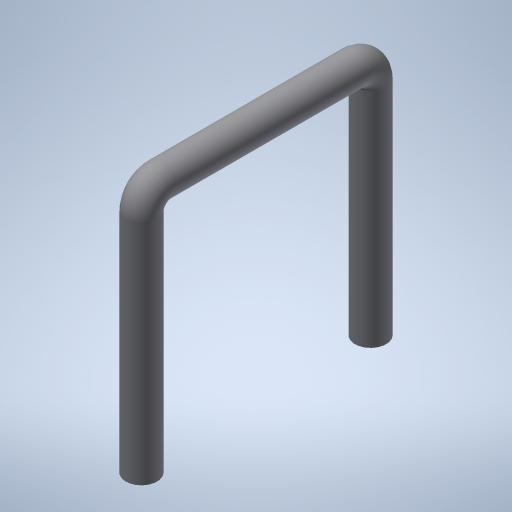
# Autodesk Inventor part: BRAZOS BAILARINA
Saved by Autodesk Inventor 2024 (Build 280153000, 153)
## iProperties
Created: 2025-03-28
Part Number: BRAZOS BAILARINA
Material: Generic
Document SubType Name: Modeling
Designer: usuario
Density: 1 g/cm^3
Appearance: Default
Author: usuario
Autodesk Inventor part; units mm, degrees
ref_plane "YZ Plane" through (0, 0, 0) normal (1, 0, 0) x (0, 1, 0)
ref_plane "XZ Plane" through (0, 0, 0) normal (0, 1, 0) x (-1, 0, 0)
ref_plane "XY Plane" through (0, 0, 0) normal (0, 0, 1) x (1, 0, 0)
sketch "Boceto1" plane through (0, 0, 0) normal (1, 0, 0) x (0, 1, 0)
  line L0 (0, 8.3393) -> (23, 8.3393)
  line L1 (25, 6.3393) -> (25, -13.2007)
  line L2 (23, -15.2007) -> (0.45, -15.2007)
  arc A0 (25, 6.3393) -> (23, 8.3393) centre (23, 6.3393) ccw
  arc A1 (23, -15.2007) -> (25, -13.2007) centre (23, -13.2007) ccw
  line L3 (0, 13.6272) -> (0, -20.4886) projected
  point P0 (0, 0)
  point P1 (25, 8.3393)
  point P2 (25, -15.2007)
  dimension "d0" = 25
  dimension "d2" = 23.54
  dimension "d6" = 2
  dimension "d8" = 24.55
  dimension "d9" = 25
  constraints: 6 end point, 4 point on circle, 4 point on line, 4 tangent, 2 centre point, 1 equal radius, 1 horizontal, 1 perpendicular, 1 vertical
  measures "d0" distance of L0.start point (25, 8.339)
  measures "d2" distance of point (25, 8.339) point (25, -15.201)
  measures "d6" radius of A0
  measures "d8" distance from line of L2.end L1
  measures "d9" distance between parallel lines of L3 L1
sketch "Boceto2" plane through (0, 0, 0) normal (0, 1, 0) x (-1, 0, 0)
  circle A0 centre (0, 8.2018) radius 1.59
  point P0 (0, 0)
  dimension "d3" = 3.18
  constraints: 1 centre point
  measures "d3" diameter of A0
sweep "Barrido1" add profiles "Boceto2" path "Boceto1" path curves L0 A0 L1 A1 L2
